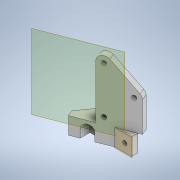
# Autodesk Inventor part: jc_conn_1
Saved by Autodesk Inventor 2020 (Build 240168000, 168)
## iProperties
Created: 2021-02-18
Part Number: jc_conn_1
Material: Generic
Document SubType Name: Modeling
Designer: Shuang Peng
Density: 1 g/cm^3
Appearance: Default
Author: Shuang Peng
Autodesk Inventor part; units mm, degrees
ref_plane "YZ Plane" through (0, 0, 0) normal (1, 0, 0) x (0, 1, 0)
ref_plane "XZ Plane" through (0, 0, 0) normal (0, 1, 0) x (-1, 0, 0)
ref_plane "Work Plane1" through (-20.7895, 15.2, 8.1501) normal (-0.3618889, 0, -0.9322212) x (-0.9322212, 0, 0.3618889)
sketch "Sketch2" plane through (-20.7895, 15.2, 8.1501) normal (-0.3618889, 0, -0.9322212) x (-0.9322212, 0, 0.3618889)
  circle A0 centre (-11, 0) radius 1 projected
  circle A1 centre (0, 11) radius 1 projected
  circle A2 centre (0, -11) radius 1 projected
  circle A3 centre (-11, 0) radius 3
  circle A4 centre (0, 11) radius 3
  circle A5 centre (0, -11) radius 3
  line L0 (0, 11) -> (3, 11)
  line L1 (0, -11) -> (3, -11)
  line L2 (3, -11) -> (3, 11)
  line L3 (0, 11) -> (-2.1213, 13.1213)
  line L4 (-2.1213, 13.1213) -> (-13.1213, 2.1213)
  line L5 (-13.1213, 2.1213) -> (-11, 0)
  line L6 (3, -11) -> (3, -14)
  line L7 (3, -14) -> (-14, -14)
  line L8 (-14, -14) -> (-14, 0)
  point P0 (-22.3298, -15.2)
  dimension "d6" = 6
  dimension "d4" = 6
  dimension "d5" = 6
  dimension "d7" = 3
  constraints: 18 end point, 4 point on circle, 3 coincident, 3 parallel, 2 centre point, 2 perpendicular, 1 collinear, 1 horizontal, 1 horizontal alignment, 1 tangent, 2 other
  measures "d4" diameter of A3
  measures "d5" diameter of A4
  measures "d7" distance of L1.end L6.end
extrude "Extrusion1" add sketch "Sketch2" along normal blind 3 contours A0 | L0 L3 A1 | L0 A4 L3 A1 | A1 L3 L0 | A1 L3 A4 L0 | L2 A5 L7 L8 A3 L4 A4 | A5 | L6 L7 A5 | A3 | A2
sketch "Sketch4" plane through (-23.5861, 1.2, 9.2357) normal (0, -1, 0) x (0.9322212, 0, -0.3618889)
  line L0 (25.9951, -3.0341) -> (28.4579, -2.8567) projected
  line L1 (27.3233, 0.0694) -> (28.4579, -2.8567) projected
  line L2 (27.3233, 0.0694) -> (25.3298, -0.0742) projected
  line L3 (25.3298, -0.0742) -> (6.5565, -7.362) projected
  line L4 (6.5565, -7.362) -> (-4.0222, -15.9035) projected
  line L5 (-2.8836, -18.8399) -> (-4.0222, -15.9035) projected
  line L6 (-2.8836, -18.8399) -> (8.0776, -9.9896) projected
  line L7 (8.0776, -9.9896) -> (25.9951, -3.0341) projected
  line L8 (17, 0) -> (0, 0) projected
  line L9 (0, 0) -> (0, -3) projected
  line L10 (17, -3) -> (0, -3) projected
  line L11 (17, 0) -> (17, -3) projected
  line L12 (6.5565, -7.362) -> (6.5565, 0)
  line L13 (17, 0) -> (0, 0) projected
  line L14 (25.3298, -0.0742) -> (24.2441, 2.7225)
  line L15 (24.2441, 2.7225) -> (17.2311, 0)
  line L16 (17, 0) -> (17, -3) projected
  line L17 (17, 0) -> (17.2311, 0)
  point P0 (6.5565, 0)
  dimension "d11" = 3
  constraints: 8 end point, 3 perpendicular, 2 point on line, 1 parallel
  measures "d11" distance of L2.end L14.end
ref_plane "Work Plane2" through (-35.5643, -7, -23.7485) normal (0, -1, 0) x (0.7068322, 0, -0.7073813)
extrude "Extrusion2" add sketch "Sketch4" along normal up to surface (8.2 mm away) contours L3 L12 L10 L11 L17 L15 L14 | L12 L8 L11 L10
sketch "Sketch5" plane through (-23.5861, 1.2, 9.2357) normal (0, 1, 0) x (0.9322212, 0, -0.3618889)
  line L0 (17, 0) -> (17, 3) projected
  line L1 (17.2311, 0) -> (17, 0) projected
  line L2 (24.2441, -2.7225) -> (17.2311, 0) projected
  line L3 (25.3298, 0.0742) -> (24.2441, -2.7225) projected
  line L4 (6.5565, 7.362) -> (25.3298, 0.0742) projected
  line L5 (6.5565, 3) -> (6.5565, 7.362) projected
  line L6 (17, 3) -> (6.5565, 3) projected
  line L7 (24.2441, -2.7225) -> (17.2311, 0) projected
  line L8 (24.2441, -2.7225) -> (24.2139, -2.8004)
  line L9 (24.2139, -2.8004) -> (17, 0)
  point P0 (25.3298, 0.0742)
  constraints: 4 end point, 1 parallel, 1 perpendicular
extrude "Extrusion3" add sketch "Sketch5" against normal up to surface (8.2 mm away) contours L1 L2 L8 L9
sketch "Sketch6" plane through (-24.6718, 1.2, 6.4391) normal (0, -1, 0) x (0.9322212, 0, -0.3618889)
  line L0 (6.5565, 0) -> (6.5565, 3) projected
  line L1 (6.5565, 3) -> (0, 3) projected
  line L2 (0, 3) -> (0, 0) projected
  line L3 (6.5565, 0) -> (0, 0) projected
  line L4 (6.5565, -4.362) -> (6.5565, 3) projected
  line L5 (6.5565, 0) -> (0, 0) projected
  line L6 (6.5565, 0) -> (6.5565, -4.362) projected
  line L7 (0, 0) -> (6.5565, -4.362)
  point P0 (25.3298, 2.9258)
  constraints: 2 end point
extrude "Extrusion4" add sketch "Sketch6" along normal up to surface (8.2 mm away)
sketch "Sketch7" plane through (0, -7, 0) normal (0, 0, -1) x (-1, 0, 0)
  circle A0 centre (3.0691, 4) radius 1.6 projected
  circle A1 centre (17.0691, 4) radius 1.6 projected
  circle A2 centre (3.0691, 4) radius 1.6 projected
  line L0 (20.1383, 8) -> (0, 8) projected
  line L1 (20.1383, 8) -> (20.1383, 0) projected
  line L2 (0, 0) -> (20.1383, 0) projected
  line L3 (0, 8) -> (0, 0) projected
  circle A3 centre (3.0691, 4) radius 1
  circle A4 centre (17.0691, 4) radius 1
  point P0 (0, 7)
  dimension "d21" = 2
  dimension "d22" = 2
  constraints: 2 centre point, 2 coincident
  measures "d21" diameter of A3
  measures "d22" diameter of A4
extrude "Extrusion5" cut sketch "Sketch7" against normal blind 10 contours A3 | A4
ref_plane "Work Plane3" through (-7.7384, 1.2, 3.0836) normal (0, 0, 1) x (1, 0, 0)
sketch "Sketch8" plane through (-7.7384, 1.2, 3.0836) normal (0, 0, 1) x (1, 0, 0)
  circle A0 centre (-9.3308, -4.2) radius 1 projected
  line L0 (-9.3308, -4.2) -> (-9.3308, -11.2) construction
  line L1 (-11.8308, -4.2) -> (-11.8308, -11.2)
  line L2 (-6.8308, -11.2) -> (-6.8308, -4.2)
  arc A1 (-6.8308, -4.2) -> (-11.8308, -4.2) centre (-9.3308, -4.2) ccw
  arc A2 (-11.8308, -11.2) -> (-6.8308, -11.2) centre (-9.3308, -11.2) ccw
  point P0 (7.7384, -1.2)
  point P1 (-9.3308, -7.7)
  dimension "d26" = 7
  dimension "d27" = 5
  constraints: 8 end point, 4 point on circle, 4 tangent, 2 centre point, 1 midpoint, 1 parallel, 1 vertical
  measures "d26" distance of L0.start L0.end
  measures "d27" diameter of A2
extrude "Extrusion6" cut sketch "Sketch8" along normal blind 10
sketch "Sketch9" plane through (-21.8751, 15.2, 5.3534) normal (-0.3618889, 0, -0.9322212) x (-0.9322212, 0, 0.3618889)
  circle A0 centre (-11, 0) radius 1 projected
  circle A1 centre (0, 11) radius 1 projected
  circle A2 centre (0, -11) radius 1 projected
  circle A3 centre (0, -11) radius 1
  circle A4 centre (-11, 0) radius 1
  circle A5 centre (0, 11) radius 1
  point P0 (-22.3298, -15.2)
  dimension "d30" = 2
  dimension "d31" = 2
  dimension "d32" = 2
  constraints: 3 centre point, 3 coincident
  measures "d30" diameter of A3
  measures "d31" diameter of A4
  measures "d32" diameter of A5
extrude "Extrusion7" cut sketch "Sketch9" against normal blind 10
thicken "Thicken1" operation add thickness 0.2 both sides no extend neighbours yes toward (0, -1, 0) faces at (-17.878, 1.2, 2.242)
sketch "Sketch13" plane through (-21.8751, 15.2, 5.3534) normal (-0.3618889, 0, -0.9322212) x (-0.9322212, 0, 0.3618889)
  line L0 (3, -14.2) -> (3, 11) projected
  arc A0 (3, 11) -> (-2.1213, 13.1213) centre (0, 11) ccw projected
  line L1 (-2.1213, 13.1213) -> (-13.1213, 2.1213) projected
  arc A1 (-13.1213, 2.1213) -> (-14, 0) centre (-11, 0) ccw projected
  line L2 (-14, 0) -> (-14, -14.2) projected
  line L3 (-14, -14.2) -> (3, -14.2) projected
  circle A2 centre (-11, 0) radius 1 projected
  circle A3 centre (0, 11) radius 1 projected
  circle A4 centre (0, -11) radius 1 projected
  line L4 (0, -11) -> (-10, -11)
  line L5 (-11, 0) -> (-21, 0)
  line L6 (0, 11) -> (-10, 11)
  circle A5 centre (-21, 0) radius 3
  circle A6 centre (-10, -11) radius 3
  circle A7 centre (-10, 11) radius 3
  line L7 (-10, 11) -> (-10, 14)
  circle A8 centre (0, 11) radius 1 projected
  line L8 (0, 11) -> (0, 14)
  arc A9 (3, 11) -> (-2.1213, 13.1213) centre (0, 11) ccw projected
  line L9 (0, 14) -> (-10, 14)
  line L10 (-10, 11) -> (-12.1213, 13.1213)
  line L11 (-21, 0) -> (-23.1213, 2.1213)
  line L12 (-23.1213, 2.1213) -> (-12.1213, 13.1213)
  line L13 (-21, 0) -> (-24, 0)
  line L14 (-3.5565, -14.2) -> (-22.3298, -14.2) projected
  line L15 (-24, 0) -> (-24, -14.2)
  line L16 (-22.3298, -14.2) -> (-24, -14.2)
  point P0 (-22.3298, -15.2)
  dimension "d57" = 10
  dimension "d58" = 10
  dimension "d59" = 10
  dimension "d60" = 6
  dimension "d61" = 6
  dimension "d62" = 6
  constraints: 24 end point, 5 point on circle, 4 horizontal, 3 centre point, 3 coincident, 3 perpendicular, 2 point on line, 1 parallel, 1 vertical
  measures "d57" distance of L4.start L4.end
  measures "d58" distance of L5.start L5.end
  measures "d59" distance of L6.start L6.end
  measures "d60" diameter of A5
  measures "d61" diameter of A6
  measures "d62" diameter of A7
extrude "Extrusion11" add sketch "Sketch13" against normal up to surface (3 mm away) contours A0 L1 L6 A7 L9 | L14 L16 L15 A5 L5 L2 | L7 L10 A7 | A7 L6 L7 | L5 A5 L12 A7 L6 L1 A1 | A7 L10 L6 | A5 L13 L5 | L5 L11 A5 | L11 L13 A5
sketch "Sketch14" plane through (-21.8751, 15.2, 5.3534) normal (-0.3618889, 0, -0.9322212) x (-0.9322212, 0, 0.3618889)
  line L0 (3, -14.2) -> (3, 11) projected
  arc A0 (3, 11) -> (0, 14) centre (0, 11) ccw projected
  line L1 (0, 14) -> (-10, 14) projected
  arc A1 (-10, 14) -> (-12.1213, 13.1213) centre (-10, 11) ccw projected
  line L2 (-12.1213, 13.1213) -> (-23.1213, 2.1213) projected
  arc A2 (-23.1213, 2.1213) -> (-24, 0) centre (-21, 0) ccw projected
  line L3 (-24, 0) -> (-24, -14.2) projected
  line L4 (-24, -14.2) -> (-14.793, -14.2) projected
  line L5 (3, -14.2) -> (-14.793, -14.2) projected
  circle A3 centre (-11, 0) radius 1 projected
  circle A4 centre (0, 11) radius 1 projected
  circle A5 centre (0, -11) radius 1 projected
  circle A6 centre (-21, 0) radius 1
  circle A7 centre (0, -11) radius 1 projected
  line L6 (0, -11) -> (-10, -11)
  circle A8 centre (-10, -11) radius 1
  circle A9 centre (0, 11) radius 1 projected
  line L7 (0, 11) -> (-10, 11)
  circle A10 centre (-10, 11) radius 1
  point P0 (-22.3298, -15.2)
  dimension "d65" = 2
  dimension "d66" = 10
  dimension "d67" = 2
  dimension "d68" = 10
  dimension "d69" = 2
  constraints: 4 end point, 3 centre point, 3 coincident, 2 horizontal
  measures "d65" diameter of A6
  measures "d66" distance of L6.start L6.end
  measures "d67" diameter of A8
  measures "d68" distance of L7.start L7.end
  measures "d69" diameter of A10
extrude "Extrusion12" cut sketch "Sketch14" against normal blind 4 contours A6 | A8 | A10
sketch "Sketch15" plane through (-21.8751, 15.2, 5.3534) normal (-0.3618889, 0, -0.9322212) x (-0.9322212, 0, 0.3618889)
  circle A0 centre (-10, 11) radius 1 projected
  circle A1 centre (-10, -11) radius 1 projected
  circle A2 centre (-21, 0) radius 1 projected
  line L0 (3, -14.2) -> (3, 11) projected
  arc A3 (3, 11) -> (0, 14) centre (0, 11) ccw projected
  line L1 (0, 14) -> (-10, 14) projected
  arc A4 (-10, 14) -> (-12.1213, 13.1213) centre (-10, 11) ccw projected
  line L2 (-12.1213, 13.1213) -> (-23.1213, 2.1213) projected
  arc A5 (-23.1213, 2.1213) -> (-24, 0) centre (-21, 0) ccw projected
  line L3 (-24, 0) -> (-24, -14.2) projected
  line L4 (-24, -14.2) -> (-14.793, -14.2) projected
  line L5 (3, -14.2) -> (-14.793, -14.2) projected
  circle A6 centre (-11, 0) radius 1 projected
  circle A7 centre (0, 11) radius 1 projected
  circle A8 centre (0, -11) radius 1 projected
  point P0 (-22.3298, -15.2)
extrude "Extrusion13" add sketch "Sketch15" against normal up to surface (3 mm away) contours A6 | A7 | A8
sketch "Sketch16" plane through (-21.8751, 15.2, 5.3534) normal (-0.3618889, 0, -0.9322212) x (-0.9322212, 0, 0.3618889)
  circle A0 centre (-10, 11) radius 1 projected
  circle A1 centre (-10, -11) radius 1 projected
  circle A2 centre (-21, 0) radius 1 projected
  line L0 (3, -14.2) -> (3, 11) projected
  arc A3 (3, 11) -> (0, 14) centre (0, 11) ccw projected
  line L1 (0, 14) -> (-10, 14) projected
  arc A4 (-10, 14) -> (-12.1213, 13.1213) centre (-10, 11) ccw projected
  line L2 (-12.1213, 13.1213) -> (-23.1213, 2.1213) projected
  arc A5 (-23.1213, 2.1213) -> (-24, 0) centre (-21, 0) ccw projected
  line L3 (-24, 0) -> (-24, -14.2) projected
  line L4 (-24, -14.2) -> (-14.793, -14.2) projected
  line L5 (3, -14.2) -> (-14.793, -14.2) projected
  circle A6 centre (-10, 11) radius 3
  circle A7 centre (-10, 11) radius 1 projected
  line L6 (-10, 11) -> (-7, 11)
  line L7 (-7, 11) -> (-7, -14.2)
  line L8 (3, -14.2) -> (-14.793, -14.2) projected
  point P0 (-22.3298, -15.2)
  point P1 (-10, 14)
  dimension "d74" = 6
  constraints: 4 end point, 1 coincident, 1 horizontal, 1 perpendicular, 1 point on line, 3 other
extrude "Extrusion14" cut sketch "Sketch16" against normal blind 4 contours L5 L7 A6 L1 A3 L0
body "Solid1"
